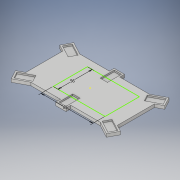
# Autodesk Inventor part: BODY_BOTTOM
Saved by Autodesk Inventor 2017 (Build 210142000, 142)
## iProperties
Created: 2017-08-24
Part Number: BODY_BOTTOM
Material: Generic
Document SubType Name: Modeling
Designer: Alexander Miller
Density: 1 g/cm^3
Appearance: Default
Author: Alexander Miller
Autodesk Inventor part; units mm, degrees
ref_plane "YZ Plane" through (0, 0, 0) normal (1, 0, 0) x (0, 1, 0)
ref_plane "XZ Plane" through (0, 0, 0) normal (0, 1, 0) x (-1, 0, 0)
ref_plane "XY Plane" through (0, 0, 0) normal (0, 0, 1) x (1, 0, 0)
sketch "Sketch1" plane through (0, 0, 0) normal (0, 1, 0) x (-1, 0, 0)
  line L0 (-75, 0) -> (75, 0) construction
  line L1 (0, 40) -> (0, -40) construction
  line L2 (75, 40) -> (56.9375, 40) construction
  line L3 (-75, 40) -> (-75, 30.3667) construction
  line L4 (-75, -40) -> (-56.9375, -40) construction
  line L5 (75, -40) -> (75, -30.3667) construction
  line L6 (349.1692, 186.2236) -> (-349.1692, -186.2236) construction
  line L7 (-349.1692, 186.2236) -> (349.1692, -186.2236) construction
  line L8 (-349.1692, 186.2236) -> (349.1692, 186.2236) construction
  line L9 (349.1692, 186.2236) -> (349.1692, -186.2236) construction
  line L10 (349.1692, -186.2236) -> (-349.1692, -186.2236) construction
  line L11 (-349.1692, -186.2236) -> (-349.1692, 186.2236) construction
  line L12 (-77.9485, 51.2059) -> (-85.9485, 36.2059)
  line L13 (-56.9375, 40) -> (-77.9485, 51.2059)
  line L14 (-75, 30.3667) -> (-85.9485, 36.2059)
  line L15 (8.5, 40) -> (8.5, 47.875)
  line L16 (8.5, 47.875) -> (-8.5, 47.875)
  line L17 (-8.5, 47.875) -> (-8.5, 40)
  line L18 (77.9485, 51.2059) -> (85.9485, 36.2059)
  line L19 (77.9485, 51.2059) -> (56.9375, 40)
  line L20 (85.9485, 36.2059) -> (75, 30.3667)
  line L21 (75, -30.3667) -> (85.9485, -36.2059)
  line L22 (85.9485, -36.2059) -> (77.9485, -51.2059)
  line L23 (77.9485, -51.2059) -> (56.9375, -40)
  line L24 (8.5, -40) -> (8.5, -47.875)
  line L25 (8.5, -47.875) -> (-8.5, -47.875)
  line L26 (-8.5, -47.875) -> (-8.5, -40)
  line L27 (-56.9375, -40) -> (-77.9485, -51.2059)
  line L28 (-77.9485, -51.2059) -> (-85.9485, -36.2059)
  line L29 (-85.9485, -36.2059) -> (-75, -30.3667)
  ellipse E0 centre (0, 0) end of major axis (-200.7823, 0) minor radius 47.875 construction
  line L30 (56.9375, 40) -> (8.5, 40)
  line L31 (8.5, 40) -> (-8.5, 40) construction
  line L32 (-8.5, 40) -> (-56.9375, 40)
  line L33 (-56.9375, 40) -> (-75, 40) construction
  line L34 (-75, 30.3667) -> (-75, -30.3667)
  line L35 (-75, -30.3667) -> (-75, -40) construction
  line L36 (-8.5, -40) -> (8.5, -40) construction
  line L37 (-56.9375, -40) -> (-8.5, -40)
  line L38 (56.9375, -40) -> (75, -40) construction
  line L39 (8.5, -40) -> (56.9375, -40)
  line L40 (75, 30.3667) -> (75, 40) construction
  line L41 (75, -30.3667) -> (75, 30.3667)
  point P0 (-81.9485, 43.7059)
  point P1 (0, 47.875)
  point P2 (81.9485, -43.7059)
  point P3 (0, -47.875)
  point P4 (-81.9485, -43.7059)
  point P5 (81.9485, 43.7059)
  dimension "d0" = 150
  dimension "d1" = 80
  dimension "d4" = 17
  dimension "d5" = 7.875
  dimension "d6" = 7.875
  constraints: 84 end point, 36 parallel, 33 perpendicular, 17 point on line, 13 midpoint, 9 equal length, 6 horizontal, 3 vertical, 2 coincident, 4 other
  measures "d0" distance of L0.end L0.start
  measures "d1" distance of L1.end L1.start
  measures "d4" distance of L15.end L16.end
  measures "d5" distance from line of L5.start L22
  measures "d6" distance between parallel lines of L31 L16
extrude "Extrusion1" add sketch "Sketch1" along normal blind 5
sketch "Sketch2" plane through (0, 5, 0) normal (0, 1, 0) x (1, 0, 0)
  line L0 (-76.9191, 47.8235) -> (-56.625, 37)
  line L1 (-56.625, 37) -> (-62.2721, 26.4118)
  line L2 (-62.2721, 26.4118) -> (-82.5662, 37.2353)
  line L3 (-82.5662, 37.2353) -> (-76.9191, 47.8235)
  line L4 (-77.9485, 51.2059) -> (-85.9485, 36.2059) projected
  line L5 (-81.9485, 43.7059) -> (0, 0) construction
  line L6 (-66.7721, 42.4118) -> (-65.5956, 44.6176) construction
  line L7 (-56.9375, 40) -> (-77.9485, 51.2059) construction
  line L8 (-81.9485, 43.7059) -> (-79.7426, 42.5294) construction
  line L9 (-6, 45.375) -> (6, 45.375)
  line L10 (6, 45.375) -> (6, 22.375)
  line L11 (6, 22.375) -> (-6, 22.375)
  line L12 (-6, 22.375) -> (-6, 45.375)
  line L13 (8.5, 47.875) -> (-8.5, 47.875) projected
  line L14 (0, 47.875) -> (0, 45.375) construction
  line L15 (6, 33.875) -> (8.5, 33.875) construction
  line L16 (56.625, 37) -> (76.9191, 47.8235)
  line L17 (76.9191, 47.8235) -> (82.5662, 37.2353)
  line L18 (82.5662, 37.2353) -> (62.2721, 26.4118)
  line L19 (62.2721, 26.4118) -> (56.625, 37)
  line L20 (85.9485, 36.2059) -> (77.9485, 51.2059) projected
  line L21 (0, 0) -> (81.9485, 43.7059) construction
  line L22 (81.9485, 43.7059) -> (79.7426, 42.5294) construction
  line L23 (75, 30.3667) -> (85.9485, 36.2059) construction
  line L24 (73.5956, 29.6176) -> (72.4191, 31.8235) construction
  line L25 (-120.3279, 0) -> (120.3279, 0) construction
  line L26 (-76.9191, -47.8235) -> (-56.625, -37)
  line L27 (-56.625, -37) -> (-62.2721, -26.4118)
  line L28 (-62.2721, -26.4118) -> (-82.5662, -37.2353)
  line L29 (-82.5662, -37.2353) -> (-76.9191, -47.8235)
  line L30 (-6, -45.375) -> (6, -45.375)
  line L31 (6, -45.375) -> (6, -22.375)
  line L32 (6, -22.375) -> (-6, -22.375)
  line L33 (-6, -22.375) -> (-6, -45.375)
  line L34 (56.625, -37) -> (76.9191, -47.8235)
  line L35 (76.9191, -47.8235) -> (82.5662, -37.2353)
  line L36 (82.5662, -37.2353) -> (62.2721, -26.4118)
  line L37 (62.2721, -26.4118) -> (56.625, -37)
  dimension "d9" = 23
  dimension "d10" = 12
  constraints: 64 end point, 12 symmetric about line, 11 midpoint, 8 equal length, 8 parallel, 8 perpendicular, 3 point on line, 1 coincident, 1 horizontal, 1 vertical alignment
  measures "d9" distance between parallel lines of L1 L3
  measures "d10" distance between parallel lines of L2 L0
extrude "Extrusion2" cut sketch "Sketch2" against normal blind 2.5
sketch "Sketch3" plane through (0, 5, 0) normal (0, 1, 0) x (1, 0, 0)
  line L0 (-32.8863, -27.7762) -> (52.1137, -27.7762)
  line L1 (52.1137, -27.7762) -> (52.1137, 28.2238)
  line L2 (52.1137, 28.2238) -> (-32.8863, 28.2238)
  line L3 (-32.8863, 28.2238) -> (-32.8863, -27.7762)
  point P0 (0, 0)
  dimension "d13" = 85
  dimension "d14" = 56
  constraints: 8 end point, 2 parallel, 1 horizontal, 1 perpendicular
  measures "d13" distance of L0.start L0.end
  measures "d14" distance of L2.end L0.start
equation "\"d0\" = body_A"
equation "\"d1\" = body_B"
equation "\"d4\" = body_C"
equation "\"d5\" = body_D"
equation "\"d6\" = body_E"
equation "\"d9\" = servo_A"
equation "\"d10\" = servo_B"
equation "\"body_A\" = 150"
equation "\"body_B\" = 80"
equation "\"body_D\" = 0.25 * servo_D"
equation "\"body_E\" = 0.25 * servo_D"
equation "\"body_C\" = 17"
equation "\"servo_A\" = 23"
equation "\"servo_B\" = 12"
equation "\"servo_D\" = 31.5"
body "Solid1"
